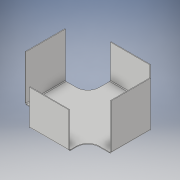
# Autodesk Inventor part: batBox
Saved by Autodesk Inventor 2017 (Build 210142000, 142)
## iProperties
Created: 2017-02-14
Part Number: batBox
Material: Generic
Document SubType Name: Sheet Metal
Designer: kingb
Density: 1 g/cm^3
Sheet Metal Rule: Default
Appearance: Default
Flat Pattern Width: 33.655 cm
Flat Pattern Length: 39.37 cm
Flat Pattern Area: 1325 cm^2
Sheet Metal Width: 13.250 in
Sheet Metal Length: 15.500 in
Sheet Metal Area: 205.375 in^2
Author: kingb
Autodesk Inventor part; units mm, degrees
ref_plane "YZ Plane" through (0, 0, 0) normal (1, 0, 0) x (0, 1, 0)
ref_plane "XZ Plane" through (0, 0, 0) normal (0, 1, 0) x (-1, 0, 0)
ref_plane "XY Plane" through (0, 0, 0) normal (0, 0, 1) x (1, 0, 0)
sketch "Sketch1" plane through (0, 0, 0) normal (0, 1, 0) x (-1, 0, 0)
  line L0 (0, 0) -> (88.9, 0)
  line L1 (88.9, 0) -> (88.9, -95.25)
  line L2 (88.9, -336.55) -> (0, -336.55)
  line L3 (0, -336.55) -> (0, -234.95)
  line L4 (-152.4, -209.55) -> (-25.4, -209.55)
  line L5 (241.3, -209.55) -> (241.3, -120.65)
  line L6 (241.3, -120.65) -> (114.3, -120.65)
  line L7 (-152.4, -120.65) -> (-152.4, -209.55)
  line L8 (88.9, -234.95) -> (88.9, -336.55)
  line L9 (0, -95.25) -> (0, 0)
  line L10 (-25.4, -120.65) -> (-152.4, -120.65)
  line L11 (114.3, -209.55) -> (241.3, -209.55)
  arc A0 (114.3, -209.55) -> (88.9, -234.95) centre (114.3, -234.95) ccw
  arc A1 (0, -234.95) -> (-25.4, -209.55) centre (-25.4, -234.95) ccw
  arc A2 (-25.4, -120.65) -> (0, -95.25) centre (-25.4, -95.25) ccw
  arc A3 (88.9, -95.25) -> (114.3, -120.65) centre (114.3, -95.25) ccw
  point P0 (88.9, -168.275)
  point P1 (88.9, -209.55)
  point P2 (88.9, -120.65)
  point P3 (0, -120.65)
  dimension "d0" = 88.9
  dimension "d1" = 336.55
  dimension "d2" = 393.7
  dimension "d3" = 41.275
  dimension "d4" = 152.4
  dimension "d5" = 88.9
  dimension "d8" = 168.275
  dimension "d9" = 47.625
  dimension "d10" = 120.65
  dimension "d11" = 127
  dimension "d12" = 209.55
  dimension "d13" = 241.3
  dimension "d14" = 25.4
  measures "d0" distance of L2.start L2.end
  measures "d1" distance of L0.end L2.start
  measures "d2" distance of L4.start L5.start
  measures "d3" distance from line of point (88.9, -168.275) L4
  measures "d4" distance from line of L1 L5.start
  measures "d5" distance of L5.start L5.end
  measures "d8" distance from line of L0 point (88.9, -168.275)
  measures "d9" distance of point (88.9, -120.65) point (88.9, -168.275)
  measures "d10" distance of L0.end point (88.9, -120.65)
  measures "d11" distance of point (88.9, -209.55) L2.start
  measures "d12" distance from line of L0 point (88.9, -209.55)
  measures "d13" distance between parallel lines of L5 L9
  measures "d14" radius of A0
extrude "Plate1" add sketch "Sketch1" along normal blind 1.5875
sketch "Sketch2" plane through (0, 1.5875, 0) normal (0, 1, 0) x (1, 0, 0)
  arc A0 (0, 234.95) -> (25.4, 209.55) centre (25.4, 234.95) ccw projected
  arc A1 (25.4, 120.65) -> (0, 95.25) centre (25.4, 95.25) ccw projected
  arc A2 (-88.9, 95.25) -> (-114.3, 120.65) centre (-114.3, 95.25) ccw projected
  arc A3 (-114.3, 209.55) -> (-88.9, 234.95) centre (-114.3, 234.95) ccw projected
  line L0 (0, 234.95) -> (0, 95.25)
  arc A4 (25.4, 120.65) -> (0, 95.25) centre (25.4, 95.25) ccw projected
  line L1 (25.4, 120.65) -> (-114.3, 120.65)
  arc A5 (-88.9, 95.25) -> (-114.3, 120.65) centre (-114.3, 95.25) ccw projected
  line L2 (-88.9, 95.25) -> (-88.9, 234.95)
  arc A6 (-114.3, 209.55) -> (-88.9, 234.95) centre (-114.3, 234.95) ccw projected
  line L3 (-114.3, 209.55) -> (25.4, 209.55)
  line L4 (-139.7, 209.55) -> (-139.7, 120.65)
  line L5 (-241.3, 209.55) -> (-114.3, 209.55) projected
  line L6 (-114.3, 120.65) -> (-241.3, 120.65) projected
  line L7 (25.4, 209.55) -> (152.4, 209.55) projected
  line L8 (50.8, 209.55) -> (50.8, 120.65)
  line L9 (152.4, 120.65) -> (25.4, 120.65) projected
  line L10 (-88.9, 260.35) -> (0, 260.35)
  line L11 (0, 336.55) -> (0, 234.95) projected
  line L12 (-88.9, 234.95) -> (-88.9, 336.55) projected
  line L13 (-88.9, 79.375) -> (0, 79.375)
  point P0 (0, 0)
  dimension "d16" = 139.7
  dimension "d17" = 139.7
  dimension "d18" = 50.8
  dimension "d19" = 0
  dimension "d20" = 0
  dimension "d21" = 50.8
  dimension "d22" = 180.975
  dimension "d23" = 50.8
  constraints: 16 end point, 5 point on line, 5 tangent, 4 perpendicular, 2 point on circle, 2 vertical, 1 horizontal, 1 parallel
  measures "d16" distance of L1.start L1.end
  measures "d17" distance of L2.start L2.end
  measures "d18" distance between parallel lines of L4 L2
  measures "d19" distance from line of L5 L4.start
  measures "d20" distance from line of L6 L4.end
  measures "d21" distance between parallel lines of L0 L8
  measures "d22" distance between parallel lines of L13 L10
  measures "d23" distance between parallel lines of L3 L10
fold "Fold1" angle 90 bend radius 1.5875 thickness 1.5875 k factor 0.44 line from (-139.7, 1.5875, -209.55) to (-139.7, 1.5875, -120.65) line at bend centre moving side (-1, 0, 0) folds toward (0, 1, 0)
fold "Fold2" angle 90 bend radius 1.5875 thickness 1.5875 k factor 0.44 line from (50.8, 1.5875, -209.55) to (50.8, 1.5875, -120.65) line at bend centre moving side (1, 0, 0) folds toward (0, 1, 0)
fold "Fold3" angle 90 bend radius 1.5875 thickness 1.5875 k factor 0.44 line from (-88.9, 1.5875, -79.375) to (0, 1.5875, -79.375) line at bend centre moving side (0, 0, 1) folds toward (0, 1, 0)
fold "Fold4" angle 90 bend radius 1.5875 thickness 1.5875 k factor 0.44 line from (-88.9, 1.5875, -260.35) to (0, 1.5875, -260.35) line at bend centre moving side (0, 0, -1) folds toward (0, 1, 0)
equation "\"d24\" = BendReliefWidth"
equation "\"d25\" = BendReliefDepth"
equation "\"d26\" = MinimumRemnant"
equation "\"d27\" = BendRadius"
equation "\"d29\" = BendRadius"
equation "\"d30\" = BendReliefWidth"
equation "\"d31\" = BendReliefDepth"
equation "\"d32\" = MinimumRemnant"
equation "\"d33\" = BendRadius"
equation "\"d35\" = BendRadius"
equation "\"d36\" = BendReliefWidth"
equation "\"d37\" = BendReliefDepth"
equation "\"d38\" = MinimumRemnant"
equation "\"d39\" = BendRadius"
equation "\"d41\" = BendRadius"
equation "\"d42\" = BendReliefWidth"
equation "\"d43\" = BendReliefDepth"
equation "\"d44\" = MinimumRemnant"
equation "\"d45\" = BendRadius"
equation "\"d47\" = BendRadius"
equation "\"BendRadius\" = Thickness"
equation "\"BendReliefWidth\" = Thickness"
equation "\"BendReliefDepth\" = 0.5 * Thickness"
equation "\"CornerReliefSize\" = 4 * Thickness"
equation "\"MinimumRemnant\" = 2 * Thickness"
equation "\"TransitionRadius\" = BendRadius"
equation "\"JacobiRadiusSize\" = Thickness"
equation "\"GapSize\" = Thickness"
equation "\"d15\" = BendRadius"
equation "\"Thickness\" = 1.5875"
body "Solid1"
